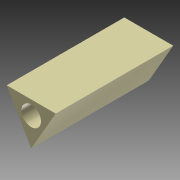
# Autodesk Inventor part: Triangle
Saved by Autodesk Inventor 2014 (Build 180170000, 170)
## iProperties
Created: 2014-03-16
Part Number: Triangle
Material: Nylon 6/6
Document SubType Name: Modeling
Designer: Pranav
Density: 1.13 g/cm^3
Appearance: Nylon 6
Mass: 26.678 g
Surface Area: 109.179 cm^2
Volume: 23.6088 cm^3
Author: Pranav
Autodesk Inventor part; units mm, degrees
ref_plane "YZ Plane" through (0, 0, 0) normal (1, 0, 0) x (0, 1, 0)
ref_plane "XZ Plane" through (0, 0, 0) normal (0, 1, 0) x (-1, 0, 0)
ref_plane "XY Plane" through (0, 0, 0) normal (0, 0, 1) x (1, 0, 0)
sketch "Sketch1" plane through (0, 0, 0) normal (0, 0, 1) x (1, 0, 0)
  circle A0 centre (0, 0) radius 6.35
  line L0 (15.875, 9.1654) -> (0, -18.3309)
  line L1 (0, -18.3309) -> (-15.875, 9.1654)
  line L2 (-15.875, 9.1654) -> (15.875, 9.1654)
  dimension "d2" = 12.7
  dimension "d3" = 31.75
  constraints: 6 end point, 3 coincident, 1 centre point, 7 other
  measures "d2" diameter of A0
  measures "d3" distance of L0.end L1.end
extrude "Extrusion1" add sketch "Sketch1" along normal blind 76.2
body "Solid1"
